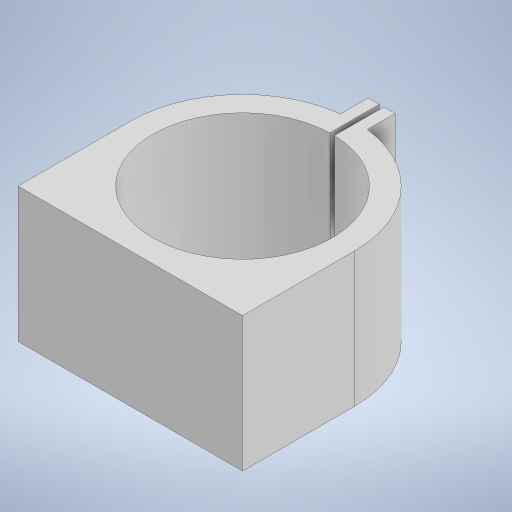
# Autodesk Inventor part: MotorClamp
Saved by Autodesk Inventor 2024 (Build 280153000, 153)
## iProperties
Created: 2023-08-28
Part Number: MotorClamp
Material: Generic
Document SubType Name: Modeling
Designer: KirikDK
Density: 1 g/cm^3
Appearance: Default
Author: KirikDK
Autodesk Inventor part; units mm, degrees
ref_plane "YZ Plane" through (0, 0, 0) normal (1, 0, 0) x (0, 1, 0)
ref_plane "XZ Plane" through (0, 0, 0) normal (0, 1, 0) x (-1, 0, 0)
ref_plane "XY Plane" through (0, 0, 0) normal (0, 0, 1) x (1, 0, 0)
sketch "Sketch1" plane through (0, 0, 0) normal (0, 1, 0) x (-1, 0, 0)
  circle A0 centre (0, 0) radius 50
  circle A1 centre (0, 0) radius 40
  line L0 (50, 0) -> (-50, 0)
  line L1 (-50, 0) -> (-50, 50)
  line L2 (-50, 50) -> (50, 50)
  line L3 (50, 50) -> (50, 0)
  line L4 (6, -46) -> (-6, -46)
  line L5 (-6, -46) -> (-6, -62)
  line L6 (-6, -62) -> (6, -62)
  line L7 (6, -62) -> (6, -46)
  line L8 (1, -64) -> (-1, -64)
  line L9 (-1, -64) -> (-1, -35)
  line L10 (-1, -35) -> (1, -35)
  line L11 (1, -35) -> (1, -64)
  point P0 (1, -39.9875)
  point P1 (1, -62)
  point P2 (6, -49.6387)
  point P3 (-6, -49.6387)
  point P4 (-1, -62)
  point P5 (-1, -39.9875)
  dimension "d0" = 100
  constraints: 24 end point, 6 parallel, 3 horizontal, 3 perpendicular, 2 coincident, 1 centre point, 3 other
extrude "Extrusion1" add sketch "Sketch1" along normal blind 60 contours L0 A1 A0 | A0 L7 L4 L11 A1 L0 | A0 L2 L3 | A0 L1 L2 | L7 L6 L11 A0 | A0 L11 L4 L7 | L0 A1 L9 L4 L5 A0 | L5 L4 L9 A0 | A0 L9 L6 L5
body "Solid1"
